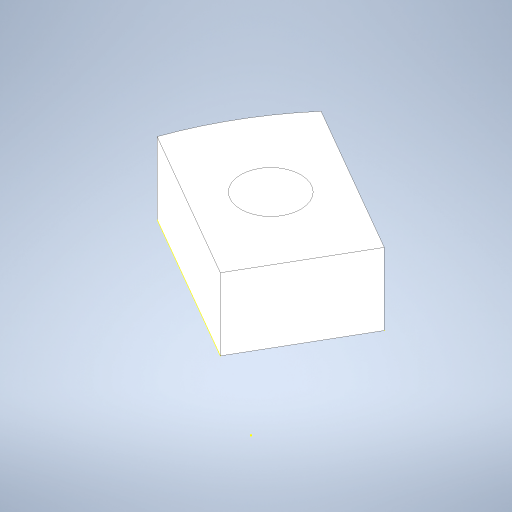
# Autodesk Inventor part: Part12
Saved by Autodesk Inventor 2024 (Build 280153000, 153)
## iProperties
Created: 2024-06-08
Part Number: Part12
Material: Generic
Document SubType Name: Sheet Metal
Designer: albah
Density: 1 g/cm^3
Sheet Metal Rule: Default_mm
Appearance: Default
Author: albah
Autodesk Inventor part; units mm, degrees
ref_plane "YZ Plane" through (0, 0, 0) normal (1, 0, 0) x (0, 1, 0)
ref_plane "XZ Plane" through (0, 0, 0) normal (0, 1, 0) x (-1, 0, 0)
ref_plane "XY Plane" through (0, 0, 0) normal (0, 0, 1) x (1, 0, 0)
sketch "Sketch7" plane through (0, 0, 0) normal (0, 1, 0) x (-1, 0, 0)
  circle A0 centre (-6.4493, -2.4672) radius 27.5
  circle A1 centre (-6.4493, -2.4672) radius 3.05
  line L0 (-6.4493, -2.4672) -> (-6.4493, 25.0328)
  line L1 (-11.4493, 39.8773) -> (-1.4493, 39.8773)
  line L2 (-1.4493, 39.8773) -> (-1.4493, 10.1882)
  line L3 (-1.4493, 10.1882) -> (-11.4493, 10.1882)
  line L4 (-11.4493, 10.1882) -> (-11.4493, 39.8773)
  line L5 (-11.4493, 39.8773) -> (-1.4493, 10.1882) construction
  line L6 (-1.4493, 39.8773) -> (-11.4493, 10.1882) construction
  line L7 (-45.6207, -19.3094) -> (-19.9093, -4.4649)
  line L8 (-19.9093, -4.4649) -> (-14.9093, -13.1251)
  line L9 (-14.9093, -13.1251) -> (-40.6207, -27.9696)
  line L10 (27.7221, -27.9696) -> (2.0107, -13.1251)
  line L11 (2.0107, -13.1251) -> (7.0107, -4.4649)
  line L12 (7.0107, -4.4649) -> (32.7221, -19.3094)
  point P0 (0, 0)
  point P1 (14.4694, -20.3182)
  point P2 (19.4694, -11.6579)
  dimension "d8" = 360
  constraints: 26 end point, 2 midpoint, 2 parallel, 1 centre point, 1 horizontal, 1 perpendicular, 1 vertical, 25 other
extrude "Extrusion2" add sketch "Sketch7" along normal blind 6 contours A0 L10 L11 L12
sketch "Sketch8" plane through (0, 6, 0) normal (0, 1, 0) x (1, 0, 0)
  arc A0 (-14.4694, 20.3182) -> (-19.4694, 11.6579) centre (6.4493, 2.4672) ccw projected
  line L0 (-19.4694, 11.6579) -> (-7.0107, 4.4649) projected
  line L1 (-14.4694, 20.3182) -> (-19.4694, 11.6579)
  circle A1 centre (-10.7401, 12.3915) radius 2.5
  point P0 (0, 0)
  dimension "d11" = 5
  constraints: 2 end point, 1 centre point, 1 perpendicular
  measures "d11" diameter of A1
extrude "Extrusion3" cut sketch "Sketch8" against normal through all contours A1
sketch "Sketch12" plane through (0, 0, 0) normal (0, -1, 0) x (1, 0, 0)
  line L0 (-2.0107, -13.1251) -> (-14.4694, -20.3182) projected
  line L1 (-19.4694, -11.6579) -> (-7.0107, -4.4649) projected
  line L2 (-14.4694, -20.3182) -> (-19.4694, -11.6579)
  point P0 (0, 0)
  constraints: 2 end point, 1 perpendicular
equation "\"BendRadius\" = Thickness"
equation "\"BendReliefWidth\" = Thickness"
equation "\"BendReliefDepth\" = 0.5 * Thickness"
equation "\"CornerReliefSize\" = 4 * Thickness"
equation "\"MinimumRemnant\" = 2 * Thickness"
equation "\"TransitionRadius\" = BendRadius"
equation "\"JacobiRadiusSize\" = BendRadius"
equation "\"GapSize\" = Thickness"
equation "\"Thickness\" = 0.5"
body "Solid2"
